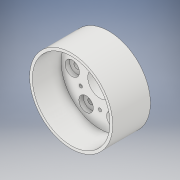
# Autodesk Inventor part: Base
Saved by Autodesk Inventor 2017 SP1 (Build 210196100, 196)
## iProperties
Created: 2017-09-22
Part Number: Base
Material: ABS Plastic
Document SubType Name: Modeling
Designer: Zach
Density: 1.06 g/cm^3
Appearance: CR White
Author: Zach
Autodesk Inventor part; units mm, degrees
ref_plane "YZ Plane" through (0, 0, 0) normal (1, 0, 0) x (0, 1, 0)
ref_plane "XZ Plane" through (0, 0, 0) normal (0, 1, 0) x (-1, 0, 0)
ref_plane "XY Plane" through (0, 0, 0) normal (0, 0, 1) x (1, 0, 0)
sketch "Sketch1" plane through (0, 0, 0) normal (0, 0, 1) x (1, 0, 0)
  circle A0 centre (0, 0) radius 37.5
  dimension "d0" = 75
  constraints: 1 centre point, 1 coincident
  measures "d0" diameter of A0
extrude "Extrusion1" add sketch "Sketch1" along normal blind 34
sketch "Sketch2" plane through (0, 0, 34) normal (0, 0, 1) x (1, 0, 0)
  circle A0 centre (0, 0) radius 37.5 projected
  circle A1 centre (0, 0) radius 35
  dimension "d105" = 70
  constraints: 1 centre point
  measures "d105" diameter of A1
extrude "Extrusion2" cut sketch "Sketch2" against normal blind 26 contours A1
sketch "Sketch3" plane through (0, 0, 8) normal (0, 0, 1) x (1, 0, 0)
  circle A0 centre (0, 0) radius 11
  dimension "d6" = 22
  constraints: 1 centre point, 1 coincident
  measures "d6" diameter of A0
extrude "Extrusion3" cut sketch "Sketch3" against normal through all
sketch "Sketch4" plane through (0, 0, 8) normal (0, 0, 1) x (1, 0, 0)
  circle A0 centre (25, 0) radius 6.5
  circle A1 centre (12.5, 21.6506) radius 6.5
  circle A2 centre (-12.5, 21.6506) radius 6.5
  circle A3 centre (-25, 0) radius 6.5
  circle A4 centre (-12.5, -21.6506) radius 6.5
  circle A5 centre (12.5, -21.6506) radius 6.5
  point P0 (0, 0)
  dimension "d9" = 13
  dimension "d10" = 25
  dimension "d13" = 360
  constraints: 6 centre point, 1 horizontal alignment, 13 other
  measures "d9" diameter of A0
  measures "d10" distance of point (0, 0) A0.centre
extrude "Extrusion4" cut sketch "Sketch4" against normal blind 4
sketch "Sketch5" plane through (0, 0, 8) normal (0, 0, 1) x (1, 0, 0)
  circle A0 centre (0, 0) radius 11 construction
  circle A1 centre (25, 0) radius 2.5
  circle A2 centre (12.5, 21.6506) radius 2.5
  circle A3 centre (-12.5, 21.6506) radius 2.5
  circle A4 centre (-25, 0) radius 2.5
  circle A5 centre (-12.5, -21.6506) radius 2.5
  circle A6 centre (12.5, -21.6506) radius 2.5
  dimension "d99" = 5
  dimension "d100" = 25
  dimension "d103" = 360
  constraints: 6 centre point, 1 coincident, 1 horizontal alignment, 13 other
  measures "d99" diameter of A1
  measures "d100" distance of A1.centre point (0, 0)
extrude "Extrusion5" cut sketch "Sketch5" against normal through all
sketch "Sketch6" plane through (0, 0, 8) normal (0, 0, 1) x (1, 0, 0)
  circle A0 centre (0, 20) radius 1.5
  circle A1 centre (-17.3205, 10) radius 1.5
  circle A2 centre (-17.3205, -10) radius 1.5
  circle A3 centre (0, -20) radius 1.5
  circle A4 centre (17.3205, -10) radius 1.5
  circle A5 centre (17.3205, 10) radius 1.5
  point P0 (0, 0)
  dimension "d24" = 3
  dimension "d25" = 20
  dimension "d28" = 360
  constraints: 6 centre point, 1 vertical alignment, 13 other
  measures "d24" diameter of A0
  measures "d25" distance of point (0, 0) A0.centre
extrude "Extrusion6" cut sketch "Sketch6" against normal through all
body "Solid1"
